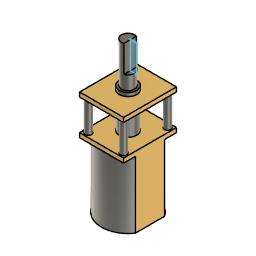
MicroMouse_Full Assembly v11 (Autodesk Fusion 360 archive; units mm, degrees)
design "Motor"
Autodesk Fusion 360 part; units mm, degrees
sketch "Sketch1" plane through (0, 0, 0) normal (0, 0, 1) x (1, 0, 0)
  circle A0 centre (0, 0) radius 6
  line L0 (-5, 6) -> (5, 6)
  line L1 (5, 6) -> (5, -6)
  line L2 (5, -6) -> (-5, -6)
  line L3 (-5, -6) -> (-5, 6)
  line L4 (-5, 6) -> (5, -6) construction
  line L5 (5, 6) -> (-5, -6) construction
  dimension "d1" = 12
  dimension "d2" = 10
  dimension "d3" = 12
  constraint coincident A0.centre origin
  constraint horizontal L0
  constraint perpendicular L0 L1
  constraint parallel L0 L2
  constraint parallel L1 L3
  constraint coincident L4 A0.centre
  constraint coincident L5 A0.centre
  measures "d1" diameter of A0
  measures "d2" distance of L1.end L2.end
  measures "d3" distance of L0.end L1.end
extrude "Extrude1" add sketch "Sketch1" along normal blind 15.1 contours A0 L1 L3
sketch "Sketch2" plane through (0, 0, 15.1) normal (0, 0, 1) x (-1, 0, 0)
  arc A0 (-5, -3.3166) -> (5, -3.3166) centre (0, 0) ccw
  line L0 (5, -3.3166) -> (5, 3.3166)
  arc A1 (5, 3.3166) -> (-5, 3.3166) centre (0, 0) ccw
  line L1 (-5, 3.3166) -> (-5, -3.3166)
  line L2 (5, -6) -> (-5, -6)
  line L3 (-5, -6) -> (-5, 6)
  line L4 (-5, 6) -> (5, 6)
  line L5 (5, 6) -> (5, -6)
  line L6 (5, -6) -> (-5, 6) construction
  line L7 (-5, -6) -> (5, 6) construction
  dimension "d6" = 10
  dimension "d7" = 12
  constraint horizontal L2
  constraint perpendicular L2 L3
  constraint parallel L2 L4
  constraint parallel L3 L5
  constraint coincident L6 A0.centre
  constraint coincident L7 A0.centre
  constraint coincident A0.centre A1.centre
  measures "d6" distance of L3.end L4.end
  measures "d7" distance of L2.end L3.end
extrude "Extrude2" add sketch "Sketch2" along normal blind 9
sketch "Sketch3" plane through (0, 0, 24.1) normal (0, 0, 1) x (-1, 0, 0)
  line L0 (5, 6) -> (-5, 6)
  line L1 (-5, 6) -> (-5, -6)
  line L2 (-5, -6) -> (5, -6)
  line L3 (5, -6) -> (5, 6)
  circle A0 centre (0, 0) radius 2
  circle A1 centre (0, 0) radius 1.5
  dimension "d10" = 4
  dimension "d11" = 3
  constraint coincident A0.centre A1.centre
  measures "d10" diameter of A0
  measures "d11" diameter of A1
extrude "Extrude3" add sketch "Sketch3" along normal blind 0.8 contours A0
extrude "Extrude4" add 1 faces at (-0.567, 0.5383, 24.1) along direction (0, 0, 1) blind 10
extrude "Extrude5" add sketch "Sketch3" along normal blind 10 contours A1
sketch "Sketch4" plane through (0, 0, 0) normal (0, 0, -1) x (1, 0, 0)
  arc A0 (-5, -3.3166) -> (5, -3.3166) centre (0, 0) ccw
  line L0 (5, -3.3166) -> (5, 3.3166)
  arc A1 (5, 3.3166) -> (-5, 3.3166) centre (0, 0) ccw
  line L1 (-5, 3.3166) -> (-5, -3.3166)
  circle A2 centre (0, 0) radius 2.5
  dimension "d18" = 5
  constraint concentric A0 A2
  measures "d18" diameter of A2
extrude "Extrude6" add sketch "Sketch4" along normal blind 1.2 contours A2
sketch "Sketch5" plane through (0, 0, 24.1) normal (0, 0, 1) x (-1, 0, 0)
  line L0 (-4, 5) -> (4, 5)
  line L1 (4, 5) -> (4, -5)
  line L2 (4, -5) -> (-4, -5)
  line L3 (-4, -5) -> (-4, 5)
  line L4 (-4, 5) -> (4, -5) construction
  line L5 (4, 5) -> (-4, -5) construction
  circle A0 centre (4, -5) radius 0.75
  circle A1 centre (-4, -5) radius 0.75
  circle A2 centre (4, 5) radius 0.75
  circle A3 centre (-4, 5) radius 0.75
  circle A4 centre (0, 0) radius 1.5
  dimension "d21" = 1.5
  dimension "d22" = 1.5
  dimension "d23" = 1.5
  dimension "d24" = 1.5
  dimension "d25" = 3
  constraint horizontal L0
  constraint perpendicular L0 L1
  constraint parallel L0 L2
  constraint parallel L1 L3
  constraint coincident L4 A4.centre
  constraint coincident L5 A4.centre
  constraint coincident A4.centre origin
  constraint coincident L1.end L2.start
  constraint coincident L2.end L3.start
  constraint coincident L0.end L1.start
  constraint coincident L0.start L3.end
  measures "d21" diameter of A0
  measures "d22" diameter of A1
  measures "d23" diameter of A2
  measures "d24" diameter of A3
  measures "d25" diameter of A4
extrude "Extrude7" cut 1 faces at (0.0498, 4.6648, 24.1) along direction (0, 0, -1) blind 7 from surface at 1
extrude "Extrude8" add sketch "Sketch5" against normal blind 8.5 contours L0 L3 A3 | L0 L3 A3 | L0 L1 A2 | L0 L1 A2 | L2 L3 A1 | L2 L3 A1 | L1 L2 A0 | L1 L2 A0 | A4
sketch "Sketch6" plane through (0, 0, 0) normal (0, 1, 0) x (1, 0, 0)
  line L0 (1, -28) -> (3, -28)
  line L1 (3, -28) -> (3, -35)
  line L2 (3, -35) -> (1, -35)
  line L3 (1, -35) -> (1, -28)
  constraint horizontal L0
  constraint vertical L1
  constraint horizontal L2
  constraint vertical L3
sketch "Sketch7" plane through (0, 0, 0) normal (0, 1, 0) x (1, 0, 0)
extrude "Extrude9" cut sketch "Sketch6" along normal blind 8
sketch "Sketch8" plane through (0, 0, 0) normal (0, 1, 0) x (1, 0, 0)
  line L0 (0.4932, -34.2266) -> (2, -34.2266)
  line L1 (2, -34.2266) -> (2, -28)
  line L2 (2, -28) -> (0.4932, -28)
  line L3 (0.4932, -28) -> (0.4932, -34.2266)
  constraint horizontal L0
  constraint vertical L1
  constraint horizontal L2
  constraint vertical L3
extrude "Extrude10" cut sketch "Sketch8" along normal blind 100
extrude "Extrude11" cut sketch "Sketch8" against normal blind 100

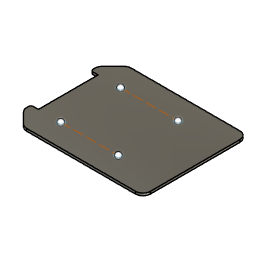
design "MicroMouse_PCB"
Autodesk Fusion 360 part; units mm, degrees
sketch "Sketch1" plane through (0, 0, 0) normal (0, 0, 1) x (1, 0, 0)
  line L0 (45, -35) -> (-45, -35)
  line L1 (-45, -35) -> (-45, 35)
  line L2 (-45, 35) -> (45, 35)
  line L3 (45, 35) -> (45, -35)
  line L4 (45, -35) -> (-45, 35) construction
  line L5 (-45, -35) -> (45, 35) construction
  dimension "d1" = 90
  dimension "d2" = 70
  constraint horizontal L0
  constraint perpendicular L0 L1
  constraint parallel L0 L2
  constraint parallel L1 L3
  constraint coincident L4 origin
  constraint coincident L5 origin
  measures "d1" distance of L1.end L2.end
  measures "d2" distance of L0.end L1.end
extrude "Extrude1" add sketch "Sketch1" along normal blind 1.6
fillet "Fillet1" radius 5 2 edges at (45, -35, 0.8) (45, 35, 0.8)
chamfer "Chamfer1" distance 10 angle 45 2 edges at (-45, -35, 0.8) (-45, 35, 0.8)
fillet "Fillet2" radius 5 4 edges at (-35, 35, 0.8) (-45, 25, 0.8) (-45, -25, 0.8) (-35, -35, 0.8)
sketch "Sketch2" plane through (0, 0, 1.6) normal (0, 0, 1) x (-1, 0, 0)
  arc A0 (36.4645, 33.5355) -> (32.9289, 35) centre (32.9289, 30) ccw
  line L0 (32.9289, 35) -> (-40, 35)
  arc A1 (-40, 35) -> (-45, 30) centre (-40, 30) ccw
  line L1 (-45, 30) -> (-45, -30)
  arc A2 (-45, -30) -> (-40, -35) centre (-40, -30) ccw
  line L2 (-40, -35) -> (32.9289, -35)
  arc A3 (32.9289, -35) -> (36.4645, -33.5355) centre (32.9289, -30) ccw
  line L3 (36.4645, -33.5355) -> (43.5355, -26.4645)
  arc A4 (43.5355, -26.4645) -> (45, -22.9289) centre (40, -22.9289) ccw
  line L4 (45, -22.9289) -> (45, 22.9289)
  arc A5 (45, 22.9289) -> (43.5355, 26.4645) centre (40, 22.9289) ccw
  line L5 (43.5355, 26.4645) -> (36.4645, 33.5355)
  line L6 (-25, -20) -> (25, -20)
  line L7 (25, -20) -> (25, 20)
  line L8 (25, 20) -> (-25, 20)
  line L9 (-25, 20) -> (-25, -20)
  line L10 (-25, -20) -> (25, 20) construction
  line L11 (25, -20) -> (-25, 20) construction
  circle A6 centre (25, 20) radius 1.75
  circle A7 centre (25, -20) radius 1.75
  dimension "d10" = 50
  dimension "d11" = 40
  dimension "d12" = 3.5
  dimension "d13" = 3.5
  constraint horizontal L6
  constraint perpendicular L6 L7
  constraint parallel L6 L8
  constraint parallel L7 L9
  constraint coincident L10 origin
  constraint coincident L11 origin
  constraint coincident L7.end L8.start
  constraint coincident L6.end L7.start
  measures "d10" distance of L7.end L8.end
  measures "d11" distance of L6.end L7.end
  measures "d12" diameter of A6
  measures "d13" diameter of A7
sketch "Sketch16" plane through (0, 0, 1.6) normal (0, 0, 1) x (-1, 0, 0)
  line L0 (25, 20) -> (-13.5, 20) construction
  line L1 (25, -20) -> (-13.5, -20) construction
  dimension "d32" = 38.5
  dimension "d33" = 38.5
  constraint horizontal L0
  constraint horizontal L1
  measures "d32" distance of L0.start L0.end
  measures "d33" distance of L1.start L1.end
sketch "Sketch17" plane through (0, 0, 1.6) normal (0, 0, 1) x (1, 0, 0)
  circle A0 centre (-25, 20) radius 1.8
  circle A1 centre (13.5, 20) radius 1.8
  circle A2 centre (-25, -20) radius 1.8
  circle A3 centre (13.5, -20) radius 1.8
  dimension "d34" = 3.6
  dimension "d35" = 3.6
  dimension "d36" = 3.6
  dimension "d37" = 3.6
  measures "d34" diameter of A0
  measures "d35" diameter of A1
  measures "d36" diameter of A2
  measures "d37" diameter of A3
extrude "Extrude7" cut sketch "Sketch17" against normal blind 4 contours A2
extrude "Extrude8" cut sketch "Sketch17" against normal blind 5 contours A3
extrude "Extrude9" cut sketch "Sketch17" against normal blind 4 contours A1
extrude "Extrude10" cut sketch "Sketch17" against normal blind 65 contours A0
sketch "Sketch18" plane through (0, 0, 1.6) normal (0, 0, 1) x (-1, 0, 0)
  circle A0 centre (25, -20) radius 1.8
  circle A1 centre (-13.5, -20) radius 1.8
  circle A2 centre (-13.5, 20) radius 1.8
  circle A3 centre (25, 20) radius 1.8
  arc A4 (36.4645, 33.5355) -> (32.9289, 35) centre (32.9289, 30) ccw
  line L0 (32.9289, 35) -> (-40, 35)
  arc A5 (-40, 35) -> (-45, 30) centre (-40, 30) ccw
  line L1 (-45, 30) -> (-45, -30)
  arc A6 (-45, -30) -> (-40, -35) centre (-40, -30) ccw
  line L2 (-40, -35) -> (32.9289, -35)
  arc A7 (32.9289, -35) -> (36.4645, -33.5355) centre (32.9289, -30) ccw
  line L3 (36.4645, -33.5355) -> (43.5355, -26.4645)
  arc A8 (43.5355, -26.4645) -> (45, -22.9289) centre (40, -22.9289) ccw
  line L4 (45, -22.9289) -> (45, 22.9289)
  arc A9 (45, 22.9289) -> (43.5355, 26.4645) centre (40, 22.9289) ccw
  line L5 (43.5355, 26.4645) -> (36.4645, 33.5355)
  line L6 (40, 20) -> (50, 20)
  line L7 (50, 20) -> (50, -20)
  line L8 (50, -20) -> (40, -20)
  line L9 (40, -20) -> (40, 20)
  line L10 (40, 20) -> (50, -20) construction
  line L11 (50, 20) -> (40, -20) construction
  point P0 (45, 0)
  dimension "d46" = 10
  constraint horizontal L6
  constraint perpendicular L6 L7
  constraint parallel L6 L8
  constraint parallel L7 L9
  constraint coincident L10 P0
  constraint coincident L11 P0
  constraint midpoint L4 P0
  measures "d46" distance of L7.end L8.end
extrude "Extrude11" cut sketch "Sketch18" against normal blind 100 contours L4 L6 L8 L9
chamfer "Chamfer4" distance 1 angle 45 2 edges at (-45, 20, 0.8) (-45, -20, 0.8)
extrude "Extrude2" [rolled back] along distance -17 taper angle 0
sketch "Sketch3" plane through (0, 0, 1.6) normal (0, 0, 1) x (-1, 0, 0)
  arc A0 (36.4645, 33.5355) -> (32.9289, 35) centre (32.9289, 30) ccw
  line L0 (32.9289, 35) -> (-40, 35)
  arc A1 (-40, 35) -> (-45, 30) centre (-40, 30) ccw
  line L1 (-45, 30) -> (-45, -30)
  arc A2 (-45, -30) -> (-40, -35) centre (-40, -30) ccw
  line L2 (-40, -35) -> (32.9289, -35)
  arc A3 (32.9289, -35) -> (36.4645, -33.5355) centre (32.9289, -30) ccw
  line L3 (36.4645, -33.5355) -> (43.5355, -26.4645)
  arc A4 (43.5355, -26.4645) -> (45, -22.9289) centre (40, -22.9289) ccw
  line L4 (45, -22.9289) -> (45, 22.9289)
  arc A5 (45, 22.9289) -> (43.5355, 26.4645) centre (40, 22.9289) ccw
  line L5 (43.5355, 26.4645) -> (36.4645, 33.5355)
  line L6 (40, -20) -> (50, -20)
  line L7 (50, -20) -> (50, 20)
  line L8 (50, 20) -> (40, 20)
  line L9 (40, 20) -> (40, -20)
  line L10 (40, -20) -> (50, 20) construction
  line L11 (50, -20) -> (40, 20) construction
  line L12 (-25, 20) -> (23.25, 20)
  arc A6 (25, 18.25) -> (23.25, 20) centre (25, 20) ccw
  line L13 (25, 18.25) -> (25, -18.25)
  arc A7 (23.25, -20) -> (25, -18.25) centre (25, -20) ccw
  line L14 (23.25, -20) -> (-25, -20)
  line L15 (-25, -20) -> (-25, 20)
  point P0 (45, 0)
  constraint horizontal L6
  constraint perpendicular L6 L7
  constraint parallel L6 L8
  constraint parallel L7 L9
  constraint coincident L10 P0
  constraint coincident L11 P0
  constraint midpoint L4 P0
extrude "Extrude3" [rolled back] along distance -20 taper angle 0
chamfer "Chamfer2" [rolled back] distance 1
chamfer "Chamfer3" [rolled back] distance 1
sketch "Sketch4" plane through (0, 0, 1.6) normal (0, 0, 1) x (-1, 0, 0)
  line L0 (45, -21) -> (44, -20)
  line L1 (44, -20) -> (40, -20)
  line L2 (40, -20) -> (40, 20)
  line L3 (40, 20) -> (44, 20)
  line L4 (44, 20) -> (45, 21)
  line L5 (45, 21) -> (45, 22.9289)
  arc A0 (45, 22.9289) -> (43.5355, 26.4645) centre (40, 22.9289) ccw
  line L6 (43.5355, 26.4645) -> (36.4645, 33.5355)
  arc A1 (36.4645, 33.5355) -> (32.9289, 35) centre (32.9289, 30) ccw
  line L7 (32.9289, 35) -> (-40, 35)
  arc A2 (-40, 35) -> (-45, 30) centre (-40, 30) ccw
  line L8 (-45, 30) -> (-45, -30)
  arc A3 (-45, -30) -> (-40, -35) centre (-40, -30) ccw
  line L9 (-40, -35) -> (32.9289, -35)
  arc A4 (32.9289, -35) -> (36.4645, -33.5355) centre (32.9289, -30) ccw
  line L10 (36.4645, -33.5355) -> (43.5355, -26.4645)
  arc A5 (43.5355, -26.4645) -> (45, -22.9289) centre (40, -22.9289) ccw
  line L11 (45, -22.9289) -> (45, -21)
  line L12 (-25, 20) -> (23.25, 20)
  arc A6 (25, 18.25) -> (23.25, 20) centre (25, 20) ccw
  line L13 (25, 18.25) -> (25, -18.25)
  arc A7 (23.25, -20) -> (25, -18.25) centre (25, -20) ccw
  line L14 (23.25, -20) -> (-25, -20)
  line L15 (-25, -20) -> (-25, 20)
sketch "Sketch5" plane through (0, 0, 1.6) normal (0, 0, 1) x (-1, 0, 0)
sketch "Sketch6" plane through (0, 0, 1.6) normal (0, 0, 1) x (-1, 0, 0)
sketch "Sketch7" plane through (0, 0, 1.6) normal (0, 0, 1) x (-1, 0, 0)
  line L0 (-45, -20) -> (-13.5, -20) construction
  dimension "d22" = 31.5
  constraint horizontal L0
  measures "d22" distance of L0.start L0.end
sketch "Sketch8" plane through (0, 0, 1.6) normal (0, 0, 1) x (-1, 0, 0)
  circle A0 centre (-13.5, -20) radius 1.8
  dimension "d23" = 3.6
  measures "d23" diameter of A0
sketch "Sketch9" plane through (0, 0, 1.6) normal (0, 0, 1) x (-1, 0, 0)
  line L0 (-45, 20) -> (-13.5, 20) construction
  dimension "d24" = 31.5
  constraint horizontal L0
  measures "d24" distance of L0.start L0.end
sketch "Sketch10" plane through (0, 0, 1.6) normal (0, 0, 1) x (-1, 0, 0)
  circle A0 centre (-13.5, 20) radius 1.8
  dimension "d25" = 3.6
  measures "d25" diameter of A0
extrude "Extrude4" [rolled back] along distance -100 taper angle 0
sketch "Sketch11" plane through (0, 0, 1.6) normal (0, 0, 1) x (-1, 0, 0)
  line L0 (45, -21) -> (44, -20)
  line L1 (44, -20) -> (40, -20)
  line L2 (40, -20) -> (40, 20)
  line L3 (40, 20) -> (44, 20)
  line L4 (44, 20) -> (45, 21)
  line L5 (45, 21) -> (45, 22.9289)
  arc A0 (45, 22.9289) -> (43.5355, 26.4645) centre (40, 22.9289) ccw
  line L6 (43.5355, 26.4645) -> (36.4645, 33.5355)
  arc A1 (36.4645, 33.5355) -> (32.9289, 35) centre (32.9289, 30) ccw
  line L7 (32.9289, 35) -> (-40, 35)
  arc A2 (-40, 35) -> (-45, 30) centre (-40, 30) ccw
  line L8 (-45, 30) -> (-45, -30)
  arc A3 (-45, -30) -> (-40, -35) centre (-40, -30) ccw
  line L9 (-40, -35) -> (32.9289, -35)
  arc A4 (32.9289, -35) -> (36.4645, -33.5355) centre (32.9289, -30) ccw
  line L10 (36.4645, -33.5355) -> (43.5355, -26.4645)
  arc A5 (43.5355, -26.4645) -> (45, -22.9289) centre (40, -22.9289) ccw
  line L11 (45, -22.9289) -> (45, -21)
  line L12 (-25, -20) -> (-2.3042, 31.9513) construction
  arc A6 (-15.3, -20) -> (-11.7, -20) centre (-13.5, -20) ccw
  line L13 (-15.3, -20) -> (-25, -20)
  line L14 (-25, -20) -> (-25, 20)
  line L15 (-25, 20) -> (-15.3, 20)
  arc A7 (-11.7, 20) -> (-15.3, 20) centre (-13.5, 20) ccw
  line L16 (-11.7, 20) -> (23.25, 20)
  arc A8 (25, 18.25) -> (23.25, 20) centre (25, 20) ccw
  line L17 (25, 18.25) -> (25, -18.25)
  arc A9 (23.25, -20) -> (25, -18.25) centre (25, -20) ccw
  line L18 (23.25, -20) -> (-11.7, -20)
sketch "Sketch12" plane through (0, 0, 1.6) normal (0, 0, 1) x (-1, 0, 0)
  line L0 (-13.5111, -20.0267) -> (-13.5111, -35)
  line L1 (-13.5111, -35) -> (-13.5111, -20.0267)
  constraint vertical L0
extrude "Extrude5" [rolled back] along distance 0.1 taper angle 0
extrude "Extrude6" [rolled back] along distance -1.6 taper angle 0
sketch "Sketch13" plane through (0, 0, 1.6) normal (0, 0, 1) x (-1, 0, 0)
  line L0 (25, 20) -> (-25, 20)
  constraint horizontal L0
sketch "Sketch14" plane through (0, 0, 1.6) normal (0, 0, 1) x (-1, 0, 0)
  line L0 (25, 20) -> (-25, 20) construction
  constraint horizontal L0
sketch "Sketch15" plane through (0, 0, 1.6) normal (0, 0, 1) x (-1, 0, 0)
  line L0 (25, 20) -> (-14, 20) construction
  line L1 (-14, 20) -> (-44, 9) construction
  constraint horizontal L0

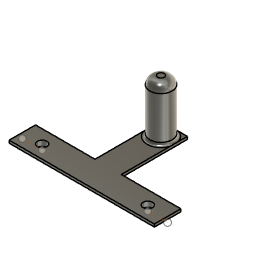
design "MicroMouse_Balance"
Autodesk Fusion 360 part; units mm, degrees
sketch "Sketch1" plane through (0, 0, 0) normal (0, 0, 1) x (1, 0, 0)
  line L0 (-27.5, 5) -> (27.5, 5)
  line L1 (27.5, 5) -> (27.5, -5)
  line L2 (27.5, -5) -> (-27.5, -5)
  line L3 (-27.5, -5) -> (-27.5, 5)
  line L4 (-27.5, 5) -> (27.5, -5) construction
  line L5 (27.5, 5) -> (-27.5, -5) construction
  dimension "d1" = 55
  dimension "d2" = 10
  constraint horizontal L0
  constraint perpendicular L0 L1
  constraint parallel L0 L2
  constraint parallel L1 L3
  constraint coincident L4 origin
  constraint coincident L5 origin
  measures "d1" distance of L1.end L2.end
  measures "d2" distance of L0.end L1.end
sketch "Sketch2" plane through (0, 0, 0) normal (0, 0, 1) x (1, 0, 0)
  line L0 (-27.5, 0) -> (-20, 0) construction
  line L1 (27.5, 0) -> (20, 0) construction
  dimension "d3" = 7.5
  dimension "d4" = 7.5
  constraint horizontal L0
  constraint horizontal L1
  measures "d3" distance of L0.start L0.end
  measures "d4" distance of L1.start L1.end
sketch "Sketch3" plane through (0, 0, 0) normal (0, 0, 1) x (1, 0, 0)
  circle A0 centre (-20, 0) radius 1.8
  circle A1 centre (20, 0) radius 1.8
  dimension "d7" = 3.6
  dimension "d8" = 3.6
  measures "d7" diameter of A0
  measures "d8" diameter of A1
extrude "Extrude1" add sketch "Sketch1" along normal blind 2
extrude "Extrude2" cut sketch "Sketch3" along normal blind 10
sketch "Sketch5" plane through (0, 5, 0) normal (0, 1, 0) x (-1, 0, 0)
  line L0 (-27.5, 0) -> (27.5, 0)
  line L1 (27.5, 0) -> (27.5, 2)
  line L2 (27.5, 2) -> (-27.5, 2)
  line L3 (-27.5, 2) -> (-27.5, 0)
  line L4 (-5, 2) -> (5, 2)
  line L5 (5, 2) -> (5, 0)
  line L6 (5, 0) -> (-5, 0)
  line L7 (-5, 0) -> (-5, 2)
  constraint horizontal L4
  constraint vertical L5
  constraint horizontal L6
  constraint vertical L7
  constraint coincident L0 L5.end
  constraint coincident L2 L4.start
extrude "Extrude3" add sketch "Sketch5" along normal blind 25 contours L0 L2 L4 L5 L6 L7
sketch "Sketch6" plane through (0, 0, 2) normal (0, 0, 1) x (-1, 0, 0)
  circle A0 centre (-20, 0) radius 1.8
  circle A1 centre (20, 0) radius 1.8
  line L0 (27.5, 5) -> (-27.5, 5)
  line L1 (-27.5, 5) -> (-27.5, -5)
  line L2 (-27.5, -5) -> (-5, -5)
  line L3 (-5, -5) -> (-5, -30)
  line L4 (-5, -30) -> (5, -30)
  line L5 (5, -30) -> (5, -5)
  line L6 (5, -5) -> (27.5, -5)
  line L7 (27.5, -5) -> (27.5, 5)
  circle A2 centre (0, -25) radius 4.2426
extrude "Extrude4" add sketch "Sketch6" along normal blind 20 contours A2
fillet "Fillet1" radius 3 1 edges at (3.9555, 26.5342, 22)
fillet "Fillet2" radius 1 1 edges at (3.9555, 23.4658, 2)
chamfer "Chamfer1" distance 1 angle 45 8 edges at (-5, 17.5, 0) (5, 17.5, 0) (0, 30, 0) (-16.25, 5, 0) (-27.5, 0, 0) (0, -5, 0) (27.5, 0, 0) (16.25, 5, 0)
